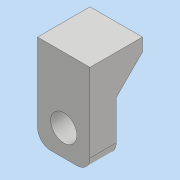
# Autodesk Inventor part: 2
Saved by Autodesk Inventor 2017 (Build 210142000, 142)
## iProperties
Part Number: 2
Material: 一般
Document SubType Name: Modeling
Designer: d8910
Density: 1 g/cm^3
Appearance: 預設
Author: d8910
Autodesk Inventor part; units mm, degrees
ref_plane "YZ Plane" through (0, 0, 0) normal (1, 0, 0) x (0, 1, 0)
ref_plane "XZ Plane" through (0, 0, 0) normal (0, 1, 0) x (-1, 0, 0)
ref_plane "XY Plane" through (0, 0, 0) normal (0, 0, 1) x (1, 0, 0)
sketch "草圖1" plane through (0, 0, 0) normal (0, 1, 0) x (-1, 0, 0)
  line L0 (10, 15) -> (-10, 15)
  line L1 (-10, 15) -> (-10, -15)
  line L2 (-5, -20) -> (5, -20)
  line L3 (10, -15) -> (10, 15)
  arc A0 (5, -20) -> (10, -15) centre (5, -15) ccw
  arc A1 (-10, -15) -> (-5, -20) centre (-5, -15) ccw
  circle A2 centre (0, -10) radius 5
  point P0 (0, 0)
  point P1 (10, -20)
  point P2 (0, -20)
  point P3 (10, 0)
  dimension "d0" = 35
  dimension "d1" = 20
  dimension "d2" = 5
  dimension "d3" = 10
  dimension "d4" = 10
  constraints: 8 end point, 4 point on circle, 4 tangent, 3 centre point, 2 midpoint, 2 parallel, 2 point on line, 2 vertical alignment, 1 equal radius, 1 horizontal, 1 horizontal alignment, 1 perpendicular
  measures "d0" distance of point (10, -20) L0.start
  measures "d1" distance of L0.start L0.end
  measures "d2" radius of A0
  measures "d3" diameter of A2
  measures "d4" distance from line of L2 A2.centre
extrude "擠出1" add sketch "草圖1" along normal blind 10
sketch "草圖2" plane through (0, 10, 0) normal (0, 1, 0) x (1, 0, 0)
  circle A0 centre (0, 10) radius 5 construction
  line L0 (-10, -15) -> (10, -15) construction
  line L1 (10, -15) -> (10, 15) construction
  arc A1 (10, 15) -> (5, 20) centre (5, 15) ccw construction
  line L2 (5, 20) -> (-5, 20) construction
  arc A2 (-5, 20) -> (-10, 15) centre (-5, 15) ccw construction
  line L3 (-10, 15) -> (-10, -15) construction
  line L4 (10, -15) -> (10, 15) projected
  line L5 (-10, -15) -> (10, -15)
  line L6 (10, -15) -> (10, -10)
  line L7 (10, -10) -> (-5, -10)
  line L8 (-10, -10.0359) -> (-10, -15)
  line L9 (-10, -15) -> (10, -15) projected
  line L10 (-10, -15) -> (-6.3427, -15)
  line L11 (-5, -10) -> (-5, 0)
  line L12 (-5, 0) -> (-10, 0)
  line L13 (-10, 0) -> (-10, -15)
  point P0 (0, 0)
  dimension "d7" = 5
  dimension "d8" = 5
  dimension "d9" = 15
  constraints: 16 end point, 4 parallel, 2 horizontal, 2 perpendicular, 1 point on line
  measures "d7" distance of L11.end L12.end
  measures "d8" distance between parallel lines of L0 L7
  measures "d9" distance between parallel lines of L9 L12
extrude "擠出2" add sketch "草圖2" along normal blind 10
sketch "草圖3" plane through (10, 0, 15) normal (1, 0, 0) x (0, 0, -1)
  line L0 (15, 10) -> (5, 10) construction
  line L1 (15, 10) -> (15, 20) construction
  line L2 (5, 20) -> (15, 20) construction
  line L3 (5, 10) -> (5, 20) construction
  line L4 (5, 10) -> (5, 20) projected
  line L5 (30, 10) -> (15, 10) projected
  line L6 (5, 20) -> (15, 10)
  line L7 (5, 10) -> (30, 10) projected
  line L8 (15, 10) -> (5, 10)
  line L9 (5, 10) -> (5, 20)
  point P0 (15, 0)
  constraints: 6 end point, 1 collinear, 1 perpendicular
extrude "擠出3" add sketch "草圖3" against normal blind 5
